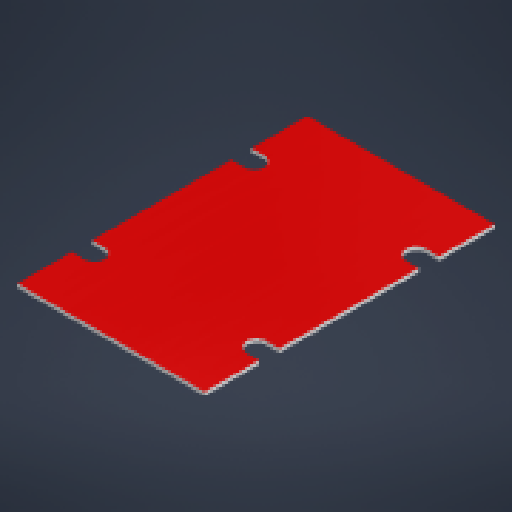
# Autodesk Inventor part: heater
Saved by Autodesk Inventor 2025 (Build 290162000, 162)
## iProperties
Created: 2024-06-24
Part Number: heater
Material: Generic
Document SubType Name: Modeling
Designer: Windows 7 was better
Density: 1 g/cm^3
Appearance: Default
Author: Windows 7 was better
Autodesk Inventor part; units mm, degrees
ref_plane "YZ Plane" through (0, 0, 0) normal (1, 0, 0) x (0, 1, 0)
ref_plane "XZ Plane" through (0, 0, 0) normal (0, 1, 0) x (-1, 0, 0)
ref_plane "XY Plane" through (0, 0, 0) normal (0, 0, 1) x (1, 0, 0)
sketch "Sketch1" plane through (0, 0, 0) normal (0, 1, 0) x (-1, 0, 0)
  line L0 (0, 0) -> (148, 0)
  line L1 (148, 0) -> (148, -229)
  line L2 (148, -229) -> (0, -229)
  line L3 (0, -229) -> (0, 0)
  line L4 (0, 0) -> (10, 0) construction
  line L5 (10, 0) -> (10, -51) construction
  circle A0 centre (10, -51) radius 8
  line L6 (10, -59) -> (0, -59)
  line L7 (10, -43) -> (0, -43)
  line L8 (10, -51) -> (10, -177) construction
  circle A1 centre (10, -177) radius 8
  line L9 (10, -169) -> (0, -169)
  line L10 (10, -185) -> (0, -185)
  line L11 (148, 0) -> (138, 0) construction
  line L12 (138, 0) -> (138, -51) construction
  circle A2 centre (138, -51) radius 8
  line L13 (138, -59) -> (148, -59)
  line L14 (138, -43) -> (148, -43)
  line L15 (138, -51) -> (138, -177) construction
  circle A3 centre (138, -177) radius 8
  line L16 (138, -185) -> (148, -185)
  line L17 (138, -169) -> (148, -169)
  dimension "d0" = 148
  dimension "d1" = 229
  dimension "d2" = 10
  dimension "d3" = 51
  dimension "d4" = 16
  dimension "d5" = 126
  dimension "d6" = 16
  dimension "d7" = 10
  dimension "d8" = 51
  dimension "d9" = 16
  constraints: 36 end point, 15 point on line, 9 perpendicular, 8 point on circle, 6 tangent, 4 centre point, 4 coincident, 3 parallel, 2 horizontal, 1 vertical
  measures "d0" distance of L1.end L2.end
  measures "d1" distance of L0.end L1.end
  measures "d2" distance of L0.start L4.end
  measures "d3" distance of L4.end L5.end
  measures "d4" diameter of A0
  measures "d5" distance of L8.start L8.end
  measures "d6" diameter of A1
  measures "d7" distance of L0.end L11.end
  measures "d8" distance of L11.end L12.end
  measures "d9" diameter of A2
extrude "Extrusion1" add sketch "Sketch1" along normal blind 3 contours L0 L1 L14 A2 L13 L17 A3 L16 L2 L3 L10 A1 L9 L6 A0 L7
body "Solid1"
